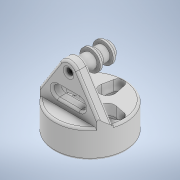
# Autodesk Inventor part: CablePlugBarb
Saved by Autodesk Inventor 2022 (Build 260153000, 153)
## iProperties
Created: 2021-10-25
Part Number: CablePlugBarb
Material: Generic
Document SubType Name: Modeling
Designer: incep
Density: 1 g/cm^3
Appearance: Default
Author: incep
Autodesk Inventor part; units mm, degrees
ref_plane "YZ Plane" through (0, 0, 0) normal (1, 0, 0) x (0, 1, 0)
ref_plane "XZ Plane" through (0, 0, 0) normal (0, 1, 0) x (-1, 0, 0)
sketch "Sketch1" plane through (0, 0, 0) normal (0, 1, 0) x (-1, 0, 0)
  circle A0 centre (0, 0) radius 16.5
  dimension "d0" = 33
  constraints: 1 centre point, 1 coincident
  measures "d0" diameter of A0
extrude "Extrusion1" add sketch "Sketch1" along normal blind 13
sketch "Sketch2" plane through (0, 0, 0) normal (0, -1, 0) x (1, 0, 0)
  line L0 (-8, 4.9075) -> (-3.75, 2.4537)
  line L1 (-3.75, 2.4537) -> (-3.75, -2.4537)
  line L2 (-3.75, -2.4537) -> (-8, -4.9075)
  line L3 (-8, -4.9075) -> (-12.25, -2.4537)
  line L4 (-12.25, -2.4537) -> (-12.25, 2.4537)
  line L5 (-12.25, 2.4537) -> (-8, 4.9075)
  line L6 (-4.9075, -8) -> (-2.4537, -3.75)
  line L7 (-2.4537, -3.75) -> (2.4537, -3.75)
  line L8 (2.4537, -3.75) -> (4.9075, -8)
  line L9 (4.9075, -8) -> (2.4537, -12.25)
  line L10 (2.4537, -12.25) -> (-2.4537, -12.25)
  line L11 (-2.4537, -12.25) -> (-4.9075, -8)
  line L12 (8, -4.9075) -> (3.75, -2.4537)
  line L13 (3.75, -2.4537) -> (3.75, 2.4537)
  line L14 (3.75, 2.4537) -> (8, 4.9075)
  line L15 (8, 4.9075) -> (12.25, 2.4537)
  line L16 (12.25, 2.4537) -> (12.25, -2.4537)
  line L17 (12.25, -2.4537) -> (8, -4.9075)
  circle A0 centre (-8, 0) radius 2.16
  circle A1 centre (0, -8) radius 2.16
  circle A2 centre (8, 0) radius 2.16
  circle A3 centre (-9.1924, -9.1924) radius 1.5
  line L18 (0, 0) -> (-9.1924, -9.1924) construction
  line L19 (0, 0) -> (-28.7343, 0) construction
  dimension "d7" = 8.5
  dimension "d8" = 8
  dimension "d9" = 180
  dimension "d10" = 4.32
  dimension "d11" = 180
  dimension "d16" = 3
  dimension "d17" = 45
  dimension "d18" = 13
  constraints: 40 end point, 4 centre point, 1 coincident, 1 horizontal, 1 horizontal alignment, 45 other
  measures "d7" distance between parallel lines of L5 L2
  measures "d8" distance of L18.start point (-8, 0)
  measures "d10" diameter of A0
  measures "d16" diameter of A3
  measures "d17" angle of L19 L18
  measures "d18" distance of L18.end point (0, 0)
extrude "Extrusion2" cut sketch "Sketch2" against normal blind 5 contours L0 L1 L2 L3 L4 L5 | L6 L7 L8 L9 L10 L11 | L12 L13 L14 L15 L16 L17 | A0 | A1 | A2
extrude "Extrusion3" cut sketch "Sketch2" against normal blind 8 contours A0 | A1 | A2
extrude "Extrusion4" cut sketch "Sketch2" against normal blind 0.5 contours A3
sketch "Sketch3" plane through (0, 13, 0) normal (0, 1, 0) x (1, 0, 0)
  circle A0 centre (-8, 0) radius 2.16 construction
  arc A1 (-8.7, -3.4293) -> (-8.7, 3.4293) centre (-8, 0) ccw
  line L0 (-8, 0) -> (-13, 0) construction
  arc A2 (-13.5, 2.4495) -> (-13.5, -2.4495) centre (-13, 0) ccw
  line L1 (-13.5, 2.4495) -> (-8.7, 3.4293)
  line L2 (-13.5, -2.4495) -> (-8.7, -3.4293)
  circle A3 centre (0, 8) radius 2.16 construction
  arc A4 (-3.4293, 8.7) -> (3.4293, 8.7) centre (0, 8) ccw
  line L3 (0, 8) -> (0, 13) construction
  arc A5 (2.4495, 13.5) -> (-2.4495, 13.5) centre (0, 13) ccw
  line L4 (2.4495, 13.5) -> (3.4293, 8.7)
  line L5 (-2.4495, 13.5) -> (-3.4293, 8.7)
  circle A6 centre (8, 0) radius 2.16 construction
  arc A7 (8.7, 3.4293) -> (8.7, -3.4293) centre (8, 0) ccw
  line L6 (8, 0) -> (13, 0) construction
  arc A8 (13.5, -2.4495) -> (13.5, 2.4495) centre (13, 0) ccw
  line L7 (13.5, -2.4495) -> (8.7, -3.4293)
  line L8 (13.5, 2.4495) -> (8.7, 3.4293)
  point P0 (0, 0)
  dimension "d21" = 8
  dimension "d22" = 4.32
  dimension "d23" = 7
  dimension "d24" = 5
  dimension "d25" = 5
  dimension "d28" = 180
  constraints: 18 end point, 12 point on circle, 9 centre point, 6 coincident, 4 tangent, 1 horizontal, 1 horizontal alignment, 29 other
  measures "d21" distance of point (0, 0) A0.centre
  measures "d22" diameter of A0
  measures "d23" diameter of A1
  measures "d24" distance of L0.start L0.end
  measures "d25" diameter of A2
extrude "Extrusion5" cut sketch "Sketch3" against normal blind 5
sketch "Sketch4" plane through (0, 13, 0) normal (0, 1, 0) x (1, 0, 0)
  line L0 (-15.7242, -5) -> (15.7242, -5)
  line L1 (13.1244, -10) -> (-13.1244, -10)
  arc A0 (-15.7242, -5) -> (-13.1244, -10) centre (0, 0) ccw
  arc A1 (13.1244, -10) -> (15.7242, -5) centre (0, 0) ccw
  dimension "d32" = 5
  dimension "d33" = 5
  constraints: 4 end point, 4 point on circle, 2 centre point, 1 coincident, 1 horizontal, 1 parallel
  measures "d32" distance from line of L0 point (0, 0)
  measures "d33" distance between parallel lines of L1 L0
extrude "Extrusion6" add sketch "Sketch4" along normal blind 20.525
ref_plane "Work Plane1" through (0, 22, 0) normal (0, 1, 0) x (1, 0, 0)
sketch "Sketch6" plane through (0, 0, 0) normal (1, 0, 0) x (0, 1, 0)
  line L0 (28.7625, 5) -> (24, 5) construction
  line L1 (24, 5) -> (24, -9) construction
  line L2 (24, -9) -> (28.7625, -9) construction
  line L3 (28.7625, -9) -> (28.7625, 5) construction
  line L4 (13, 5) -> (33.525, 5) projected
  line L5 (13, -16.5) -> (13, 5) projected
  line L6 (25.5, 0) -> (24, 0) construction
  line L7 (24, 0) -> (24, -3) construction
  line L8 (24, -3) -> (25.5, -3) construction
  line L9 (25.5, -3) -> (25.5, 0) construction
  line L10 (25.5, -3) -> (24, -3) construction
  line L11 (24, -3) -> (24, -6) construction
  line L12 (24, -6) -> (25.5, -6) construction
  line L13 (25.5, -6) -> (25.5, -3) construction
  line L14 (25.5, -6) -> (24, -6) construction
  line L15 (24, -6) -> (24, -9) construction
  line L16 (24, -9) -> (25.5, -9) construction
  line L17 (25.5, -9) -> (25.5, -6) construction
  line L18 (27.25, 5) -> (27.25, -9) construction
  line L19 (25.5, 0) -> (25.5, 5) construction
  line L20 (25.5, 5) -> (25.5, 0)
  line L21 (24, 0) -> (24, -1)
  line L22 (24, -1) -> (25.5, -3)
  line L23 (25.5, 0) -> (24, 0)
  line L24 (25.5, -3) -> (25.5, -6)
  line L25 (25.5, -6) -> (24, -6)
  line L26 (24, -6) -> (24, -7)
  line L27 (24, -7) -> (25.5, -9)
  line L28 (25.5, -9) -> (27.25, -9)
  line L29 (27.25, -9) -> (27.25, 5)
  line L30 (27.25, 5) -> (25.5, 5)
  point P0 (0, 0)
  dimension "d75" = 11
  dimension "d76" = 4.7625
  dimension "d79" = 1.5
  dimension "d80" = 3
  dimension "d81" = 5
  dimension "d83" = 1.75
  dimension "d84" = 1
  dimension "d85" = 1
  constraints: 58 end point, 8 parallel, 8 perpendicular, 8 point on line, 7 collinear, 5 horizontal, 1 vertical
  measures "d75" distance between parallel lines of L5 L1
  measures "d76" distance of L1.end L2.end
  measures "d79" distance of L7.end L8.end
  measures "d80" distance of L6.end L7.end
  measures "d81" distance between parallel lines of L6 L0
  measures "d83" distance between parallel lines of L17 L18
  measures "d84" distance of L6.end L21.end
  measures "d85" distance of L14.end L26.end
revolve "Revolution1" add sketch "Sketch6" angle 360 about axis through (0, 28.7625, -9) along (0, 0, 1)
sketch "Sketch7" plane through (15.7242, 13, 5) normal (0, 0, -1) x (-1, 0, 0)
  arc A0 (19.7373, 18.3269) -> (11.7111, 18.3269) centre (15.7242, 15.7625) ccw
  line L0 (32.2242, 0) -> (-0.7758, 0) projected
  line L1 (0, 0) -> (0, 20.525) projected
  line L2 (31.4484, 0) -> (0, 0) projected
  line L3 (0, 0) -> (31.4484, 0)
  line L4 (31.4484, 0) -> (19.7373, 18.3269)
  line L5 (0, 0) -> (11.7111, 18.3269)
  line L6 (0, 0) -> (0, 20.525)
  line L7 (31.4484, 0) -> (31.4484, 20.525) projected
  line L8 (0, 20.525) -> (31.4484, 20.525)
  line L9 (31.4484, 20.525) -> (31.4484, 0)
  circle A1 centre (15.7242, 15.7625) radius 1.5125
  line L10 (10.7242, 8) -> (20.7242, 8)
  line L11 (20.7242, 3) -> (10.7242, 3)
  arc A2 (20.7242, 3) -> (20.7242, 8) centre (20.7242, 5.5) ccw
  arc A3 (10.7242, 8) -> (10.7242, 3) centre (10.7242, 5.5) ccw
  point P0 (15.7242, -13)
  point P1 (15.7242, 0)
  point P2 (15.7242, 20.525)
  point P3 (15.7242, 3)
  point P4 (15.7242, 0)
  dimension "d22" = 4.32
  dimension "d87" = 9.525
  dimension "d89" = 11
  dimension "d94" = 5
  dimension "d96" = 3
  dimension "d97" = 10
  constraints: 16 end point, 6 point on circle, 4 centre point, 4 tangent, 3 midpoint, 2 horizontal, 2 parallel, 2 perpendicular, 2 vertical alignment, 1 coincident, 1 vertical
  measures "d87" diameter of A0
  measures "d89" distance edge to line of A0 L0
  measures "d94" distance between parallel lines of L11 L10
  measures "d96" distance of point (15.724, 0) point (15.724, 3)
  measures "d97" distance of L11.start L11.end
extrude "Extrusion7" cut sketch "Sketch7" against normal blind 20.525 contours A0 L8 L7 L4 | A0 L5 L1 L8
extrude "Extrusion8" cut sketch "Sketch7" against normal blind 20.525 contours A1
extrude "Extrusion9" cut sketch "Sketch7" against normal blind 20.525 contours L10 A2 L11 A3
fillet "Fillet1" radius 1 19 edges at (16.5, 0, 0) (2.5299, 13, -16.3049) (-16.3049, 13, 2.5299) (0, 33.525, 5) (-9.8687, 22.1635, 5) (9.8687, 22.1635, 5) (0, 33.525, 10) (-8.5688, 24.1977, 10) (8.5688, 24.1977, 10) (0, 13, 16.5) (-7.5, 18.5, 5) (0, 16, 5) (7.5, 18.5, 5) (0, 21, 5) (7.5, 18.5, 10) (0, 16, 10) (-7.5, 18.5, 10) (0, 21, 10) (1.5125, 28.7625, 10)
body "Solid1"
